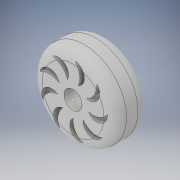
# Autodesk Inventor part: wheel
Saved by Autodesk Inventor 2019 (Build 230136000, 136)
## iProperties
Created: 2019-04-09
Part Number: wheel
Material: Ogólny
Document SubType Name: Modeling
Designer: terg
Density: 1 g/cm^3
Appearance: Domyślna
Author: terg
## iProperties of the stored document wheel_Drukowanie 3D.ipt
Created: 2019-04-09
Part Number: wheel_Drukowanie 3D
Material: Ogólny
Document SubType Name: Modeling
Designer: terg
Density: 1 g/cm^3
Appearance: Domyślna
Author: terg
Autodesk Inventor part; units mm, degrees
ref_plane "YZ Plane" through (0, 0, 0) normal (1, 0, 0) x (0, 1, 0)
ref_plane "XZ Plane" through (0, 0, 0) normal (0, 1, 0) x (-1, 0, 0)
ref_plane "XY Plane" through (0, 0, 0) normal (0, 0, 1) x (1, 0, 0)
sketch "Szkic1" plane through (0, 0, 0) normal (0, 0, 1) x (1, 0, 0)
  circle A0 centre (0, 0) radius 7.45
  dimension "d0" = 14.9
  constraints: 1 centre point, 1 coincident
  measures "d0" diameter of A0
extrude "Wyciągnięcie proste1" add sketch "Szkic1" along normal blind 6
sketch "Szkic2" plane through (0, 0, 6) normal (0, 0, 1) x (1, 0, 0)
  circle A0 centre (0, 0) radius 1.6
  dimension "d3" = 3.2
  constraints: 1 centre point, 1 coincident
  measures "d3" diameter of A0
extrude "Wyciągnięcie proste2" cut sketch "Szkic2" against normal blind 6
sketch "Szkic3" plane through (0, 0, 6) normal (0, 0, 1) x (1, 0, 0)
  point P0 (0, 0)
sketch "Szkic4" plane through (0, 0, 6) normal (0, 0, 1) x (1, 0, 0)
  circle A0 centre (0, 0) radius 1.6 construction
  arc A1 (0, -2.8) -> (1.725, -5.7878) centre (1.2407, -4.0755) ccw
  arc A2 (0, -2.8) -> (1.725, -5.7878) centre (2.9881, -3.0667) ccw
  dimension "d7" = 3.45
  dimension "d9" = 3
  constraints: 6 point on circle, 2 centre point
  measures "d7" distance of A1.start A1.end
  measures "d9" radius of A2
extrude "Wyciągnięcie proste3" cut sketch "Szkic4" against normal blind 6
pattern_circular "Szyk kołowy1" count 9 over 360 about axis through (0, 0, 6) along (0, 0, -1) of "Wyciągnięcie proste3"
fillet "Zaokrąglenie1" radius 2 2 edges at (-7.45, 0, 6) (-7.45, 0, 0)
